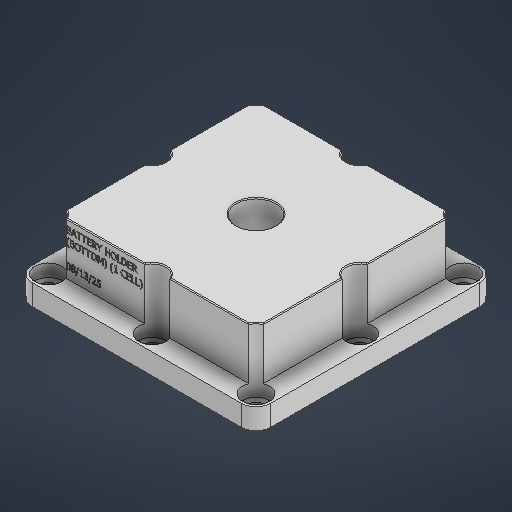
# Autodesk Inventor part: Battery Holder
Saved by Autodesk Inventor 2025 (Build 290162000, 162)
## iProperties
Created: 2025-08-08
Part Number: Battery Holder
Material: Generic
Document SubType Name: Modeling
Designer: mayhe
Density: 1 g/cm^3
Appearance: Default
Author: mayhe
Autodesk Inventor part; units mm, degrees
ref_plane "YZ Plane" through (0, 0, 0) normal (1, 0, 0) x (0, 1, 0)
ref_plane "XZ Plane" through (0, 0, 0) normal (0, 1, 0) x (-1, 0, 0)
ref_plane "XY Plane" through (0, 0, 0) normal (0, 0, 1) x (1, 0, 0)
sketch "Sketch1" plane through (0, 0, 0) normal (0, 1, 0) x (-1, 0, 0)
  line L0 (57.5, 57.5) -> (-57.5, 57.5)
  line L1 (-57.5, 57.5) -> (-57.5, -57.5)
  line L2 (-57.5, -57.5) -> (57.5, -57.5)
  line L3 (57.5, -57.5) -> (57.5, 57.5)
  line L4 (57.5, 57.5) -> (-57.5, -57.5) construction
  line L5 (-57.5, 57.5) -> (57.5, -57.5) construction
  point P0 (0, 0)
  dimension "d0" = 115
  dimension "d1" = 115
  constraints: 12 end point, 2 midpoint, 2 parallel, 1 horizontal, 1 perpendicular
  measures "d0" distance of L2.end L1.end
  measures "d1" distance of L1.end L0.end
extrude "Extrusion1" add sketch "Sketch1" along normal blind 10
sketch "Sketch4" plane through (0, 10, 0) normal (0, 1, 0) x (1, 0, 0)
  line L0 (-47.5, -47.5) -> (47.5, -47.5)
  line L1 (47.5, -47.5) -> (47.5, 47.5)
  line L2 (47.5, 47.5) -> (-47.5, 47.5)
  line L3 (-47.5, 47.5) -> (-47.5, -47.5)
  line L4 (-57.5, 57.5) -> (-57.5, -57.5) projected
  line L5 (-57.5, 0) -> (-47.5, 0)
  circle A0 centre (0, 0) radius 9.5
  point P0 (47.3285, -94.6135)
  point P1 (-53.5957, 219.1108)
  dimension "d48" = 95
  dimension "d49" = 95
  dimension "d180" = 19
  constraints: 10 end point, 2 midpoint, 2 parallel, 1 centre point, 1 horizontal, 1 perpendicular
  measures "d48" distance of L2.end L1.end
  measures "d49" distance of L1.end L0.end
  measures "d180" diameter of A0
extrude "Extrusion2" add sketch "Sketch4" along normal blind 25
sketch "Sketch5" plane through (0, 35, 0) normal (0, 1, 0) x (1, 0, 0)
  line L0 (50, 50) -> (-50, 50)
  line L1 (-50, 50) -> (-50, -50)
  line L2 (-50, -50) -> (50, -50)
  line L3 (50, -50) -> (50, 50)
  line L4 (50, 50) -> (-50, -50) construction
  line L5 (-50, 50) -> (50, -50) construction
  circle A0 centre (-50, -50) radius 3.5
  circle A1 centre (0, -50) radius 3.5
  circle A2 centre (-50, 0) radius 3.5
  circle A3 centre (0, 0) radius 3.5
  circle A4 centre (50, -50) radius 3.5
  circle A5 centre (50, 0) radius 3.5
  circle A6 centre (-50, 50) radius 3.5
  circle A7 centre (0, 50) radius 3.5
  circle A8 centre (50, 50) radius 3.5
  point P0 (0, 0)
  dimension "d156" = 100
  dimension "d157" = 100
  dimension "d158" = 7
  dimension "d161" = 50
  dimension "d164" = 50
  constraints: 12 end point, 9 centre point, 2 horizontal, 2 midpoint, 2 parallel, 1 coincident, 1 perpendicular, 1 vertical, 16 other
  measures "d156" distance of L2.end L1.end
  measures "d157" distance of L1.end L0.end
  measures "d158" diameter of A0
  measures "d161" distance of A0.centre A1.centre
  measures "d164" distance of A0.centre A2.centre
hole "Hole3" at (-50, 35, 50) at (50, 35, 50) at (-50, 35, -50) at (50, 35, -50) at (-50, 35, 0) at (0, 35, 50) at (50, 35, 0) at (0, 35, -50) direction (0, -1, 0) diameter 7.125 end through all counterbore diameter 13 counterbore depth 31
fillet "Fillet1" radius 7.125 4 edges at (57.5, 5, 57.5) (57.5, 5, -57.5) (-57.5, 5, 57.5) (-57.5, 5, -57.5)
chamfer "Chamfer1" distance 0.4 angle 45 18 edges at (-9.5, 35, 0) (-25, 35, 47.5) (0, 35, 43.5) (25, 35, 47.5) (47.5, 35, 25) (45.4038, 35, 45.4038) (43.5, 35, 0) (47.5, 35, -25) (45.4038, 35, -45.4038) (25, 35, -47.5) (3.6056, 35, -44.5917) (-3.6056, 35, -44.5917) (-25, 35, -47.5) (-45.4038, 35, -45.4038) (-47.5, 35, -25) (-43.5, 35, 0) (-47.5, 35, 25) (-45.4038, 35, 45.4038)
sketch "Sketch6" plane through (-44, 10, 47.5) normal (0, 0, 1) x (1, 0, 0)
  line L0 (0.0452, 22.2383) -> (37.6738, 22.2383) construction
  line L1 (37.6738, 22.2383) -> (37.6738, -2.1213) construction
  line L2 (37.6738, -2.1213) -> (0.0452, -2.1213) construction
  line L3 (0.0452, -2.1213) -> (0.0452, 22.2383) construction
  spline S0 degree 2 poles (2.4213, 20.0622) (2.4213, 19.835) (2.2484, 19.4867) (2.1052, 19.3731) knots 0 0 0 1 2 2 2
  spline S1 degree 2 poles (2.1052, 19.3731) (1.9323, 19.2397) (1.5395, 19.1261) (1.2283, 19.1261) knots 0 0 0 1 2 2 2
  line L4 (1.2283, 19.1261) -> (0.3539, 19.1261)
  line L5 (0.3539, 19.1261) -> (0.3539, 22.1741)
  line L6 (0.3539, 22.1741) -> (1.1616, 22.1741)
  spline S2 degree 2 poles (1.1616, 22.1741) (1.4877, 22.1741) (1.8137, 22.1321) (1.9619, 22.0506) knots 0 0 0 1 2 2 2
  spline S3 degree 2 poles (1.9619, 22.0506) (2.1274, 21.9641) (2.2781, 21.6801) (2.2781, 21.4874) knots 0 0 0 1 2 2 2
  spline S4 degree 2 poles (2.2781, 21.4874) (2.2781, 21.2725) (2.0508, 20.9316) (1.8507, 20.8353) knots 0 0 0 1 2 2 2
  line L7 (1.8507, 20.8353) -> (1.8507, 20.8205)
  spline S5 degree 2 poles (1.8507, 20.8205) (2.1224, 20.7464) (2.4213, 20.3537) (2.4213, 20.0622) knots 0 0 0 1 2 2 2
  spline S6 degree 2 poles (1.9989, 20.0449) (1.9989, 20.2178) (1.9001, 20.4401) (1.7519, 20.5191) knots 0 0 0 1 2 2 2
  spline S7 degree 2 poles (1.7519, 20.5191) (1.6556, 20.5685) (1.4284, 20.5982) (1.2184, 20.5982) knots 0 0 0 1 2 2 2
  line L8 (1.2184, 20.5982) -> (0.759, 20.5982)
  line L9 (0.759, 20.5982) -> (0.759, 19.4719)
  line L10 (0.759, 19.4719) -> (1.0875, 19.4719)
  spline S8 degree 2 poles (1.0875, 19.4719) (1.3543, 19.4719) (1.6606, 19.5213) (1.7791, 19.6003) knots 0 0 0 1 2 2 2
  spline S9 degree 2 poles (1.7791, 19.6003) (1.8927, 19.6818) (1.9989, 19.8844) (1.9989, 20.0449) knots 0 0 0 1 2 2 2
  spline S10 degree 2 poles (1.8557, 21.4306) (1.8557, 21.5393) (1.7816, 21.7023) (1.7001, 21.7492) knots 0 0 0 1 2 2 2
  spline S11 degree 2 poles (1.7001, 21.7492) (1.6013, 21.8036) (1.3617, 21.8283) (1.1468, 21.8283) knots 0 0 0 1 2 2 2
  line L11 (1.1468, 21.8283) -> (0.759, 21.8283)
  line L12 (0.759, 21.8283) -> (0.759, 20.9366)
  line L13 (0.759, 20.9366) -> (1.2184, 20.9366)
  spline S12 degree 2 poles (1.2184, 20.9366) (1.4086, 20.9366) (1.5889, 20.9761) (1.6853, 21.0378) knots 0 0 0 1 2 2 2
  spline S13 degree 2 poles (1.6853, 21.0378) (1.7791, 21.0971) (1.8557, 21.2873) (1.8557, 21.4306) knots 0 0 0 1 2 2 2
  line L14 (2.4954, 19.1261) -> (3.5229, 22.1741)
  line L15 (3.5229, 22.1741) -> (4.0219, 22.1741)
  line L16 (4.0219, 22.1741) -> (5.0494, 19.1261)
  line L17 (5.0494, 19.1261) -> (4.6221, 19.1261)
  line L18 (4.6221, 19.1261) -> (4.3455, 19.9782)
  line L19 (4.3455, 19.9782) -> (3.1821, 19.9782)
  line L20 (3.1821, 19.9782) -> (2.9054, 19.1261)
  line L21 (2.9054, 19.1261) -> (2.4954, 19.1261)
  line L22 (4.2343, 20.324) -> (3.7625, 21.7591)
  line L23 (3.7625, 21.7591) -> (3.2932, 20.324)
  line L24 (3.2932, 20.324) -> (4.2343, 20.324)
  line L25 (6.0498, 19.1261) -> (6.0498, 21.8134)
  line L26 (6.0498, 21.8134) -> (5.0272, 21.8134)
  line L27 (5.0272, 21.8134) -> (5.0272, 22.1741)
  line L28 (5.0272, 22.1741) -> (7.4774, 22.1741)
  line L29 (7.4774, 22.1741) -> (7.4774, 21.8134)
  line L30 (7.4774, 21.8134) -> (6.4549, 21.8134)
  line L31 (6.4549, 21.8134) -> (6.4549, 19.1261)
  line L32 (6.4549, 19.1261) -> (6.0498, 19.1261)
  line L33 (8.4976, 19.1261) -> (8.4976, 21.8134)
  line L34 (8.4976, 21.8134) -> (7.475, 21.8134)
  line L35 (7.475, 21.8134) -> (7.475, 22.1741)
  line L36 (7.475, 22.1741) -> (9.9252, 22.1741)
  line L37 (9.9252, 22.1741) -> (9.9252, 21.8134)
  line L38 (9.9252, 21.8134) -> (8.9026, 21.8134)
  line L39 (8.9026, 21.8134) -> (8.9026, 19.1261)
  line L40 (8.9026, 19.1261) -> (8.4976, 19.1261)
  line L41 (10.234, 19.1261) -> (10.234, 22.1741)
  line L42 (10.234, 22.1741) -> (12.1408, 22.1741)
  line L43 (12.1408, 22.1741) -> (12.1408, 21.8134)
  line L44 (12.1408, 21.8134) -> (10.6391, 21.8134)
  line L45 (10.6391, 21.8134) -> (10.6391, 20.9786)
  line L46 (10.6391, 20.9786) -> (12.0396, 20.9786)
  line L47 (12.0396, 20.9786) -> (12.0396, 20.6179)
  line L48 (12.0396, 20.6179) -> (10.6391, 20.6179)
  line L49 (10.6391, 20.6179) -> (10.6391, 19.4867)
  line L50 (10.6391, 19.4867) -> (12.1408, 19.4867)
  line L51 (12.1408, 19.4867) -> (12.1408, 19.1261)
  line L52 (12.1408, 19.1261) -> (10.234, 19.1261)
  line L53 (14.9443, 19.1261) -> (14.4182, 19.1261)
  line L54 (14.4182, 19.1261) -> (13.4549, 20.3388)
  line L55 (13.4549, 20.3388) -> (12.9905, 20.3388)
  line L56 (12.9905, 20.3388) -> (12.9905, 19.1261)
  line L57 (12.9905, 19.1261) -> (12.5854, 19.1261)
  line L58 (12.5854, 19.1261) -> (12.5854, 22.1741)
  line L59 (12.5854, 22.1741) -> (13.3709, 22.1741)
  spline S14 degree 2 poles (13.3709, 22.1741) (13.6327, 22.1741) (13.9859, 22.1172) (14.1465, 22.0135) knots 0 0 0 1 2 2 2
  spline S15 degree 2 poles (14.1465, 22.0135) (14.307, 21.9098) (14.4923, 21.5862) (14.4923, 21.3466) knots 0 0 0 1 2 2 2
  spline S16 degree 2 poles (14.4923, 21.3466) (14.4923, 21.0131) (14.1514, 20.5611) (13.86, 20.4525) knots 0 0 0 1 2 2 2
  line L60 (13.86, 20.4525) -> (14.9443, 19.1261)
  spline S17 degree 2 poles (14.0699, 21.3145) (14.0699, 21.4479) (13.9761, 21.6529) (13.8773, 21.7196) knots 0 0 0 1 2 2 2
  spline S18 degree 2 poles (13.8773, 21.7196) (13.7908, 21.7764) (13.5611, 21.8233) (13.3931, 21.8233) knots 0 0 0 1 2 2 2
  line L61 (13.3931, 21.8233) -> (12.9905, 21.8233)
  line L62 (12.9905, 21.8233) -> (12.9905, 20.6772)
  line L63 (12.9905, 20.6772) -> (13.3462, 20.6772)
  spline S19 degree 2 poles (13.3462, 20.6772) (13.5216, 20.6772) (13.8007, 20.739) (13.897, 20.8353) knots 0 0 0 1 2 2 2
  spline S20 degree 2 poles (13.897, 20.8353) (13.9859, 20.9193) (14.0699, 21.1564) (14.0699, 21.3145) knots 0 0 0 1 2 2 2
  line L64 (17.3205, 22.1741) -> (16.2905, 20.4747)
  line L65 (16.2905, 20.4747) -> (16.2905, 19.1261)
  line L66 (16.2905, 19.1261) -> (15.8854, 19.1261)
  line L67 (15.8854, 19.1261) -> (15.8854, 20.4327)
  line L68 (15.8854, 20.4327) -> (14.8554, 22.1741)
  line L69 (14.8554, 22.1741) -> (15.3049, 22.1741)
  line L70 (15.3049, 22.1741) -> (16.0929, 20.8328)
  line L71 (16.0929, 20.8328) -> (16.8907, 22.1741)
  line L72 (16.8907, 22.1741) -> (17.3205, 22.1741)
  line L73 (21.1243, 19.1261) -> (20.7192, 19.1261)
  line L74 (20.7192, 19.1261) -> (20.7192, 20.6179)
  line L75 (20.7192, 20.6179) -> (19.3162, 20.6179)
  line L76 (19.3162, 20.6179) -> (19.3162, 19.1261)
  line L77 (19.3162, 19.1261) -> (18.9111, 19.1261)
  line L78 (18.9111, 19.1261) -> (18.9111, 22.1741)
  line L79 (18.9111, 22.1741) -> (19.3162, 22.1741)
  line L80 (19.3162, 22.1741) -> (19.3162, 20.9786)
  line L81 (19.3162, 20.9786) -> (20.7192, 20.9786)
  line L82 (20.7192, 20.9786) -> (20.7192, 22.1741)
  line L83 (20.7192, 22.1741) -> (21.1243, 22.1741)
  line L84 (21.1243, 22.1741) -> (21.1243, 19.1261)
  spline S21 degree 2 poles (23.8981, 21.8258) (24.071, 21.6232) (24.2637, 21.0304) (24.2637, 20.6501) knots 0 0 0 1 2 2 2
  spline S22 degree 2 poles (24.2637, 20.6501) (24.2637, 20.2796) (24.076, 19.6793) (23.8981, 19.4768) knots 0 0 0 1 2 2 2
  spline S23 degree 2 poles (23.8981, 19.4768) (23.7104, 19.2644) (23.2139, 19.0618) (22.915, 19.0618) knots 0 0 0 1 2 2 2
  spline S24 degree 2 poles (22.915, 19.0618) (22.6063, 19.0618) (22.1123, 19.2718) (21.932, 19.4768) knots 0 0 0 1 2 2 2
  spline S25 degree 2 poles (21.932, 19.4768) (21.7566, 19.6793) (21.5689, 20.2746) (21.5689, 20.6501) knots 0 0 0 1 2 2 2
  spline S26 degree 2 poles (21.5689, 20.6501) (21.5689, 21.0329) (21.7591, 21.6158) (21.9344, 21.8258) knots 0 0 0 1 2 2 2
  spline S27 degree 2 poles (21.9344, 21.8258) (22.1123, 22.0283) (22.6088, 22.2383) (22.915, 22.2383) knots 0 0 0 1 2 2 2
  spline S28 degree 2 poles (22.915, 22.2383) (23.2263, 22.2383) (23.7252, 22.0209) (23.8981, 21.8258) knots 0 0 0 1 2 2 2
  spline S29 degree 2 poles (23.8413, 20.6501) (23.8413, 20.9514) (23.7104, 21.4182) (23.5918, 21.5714) knots 0 0 0 1 2 2 2
  spline S30 degree 2 poles (23.5918, 21.5714) (23.4708, 21.7295) (23.1299, 21.8875) (22.9175, 21.8875) knots 0 0 0 1 2 2 2
  spline S31 degree 2 poles (22.9175, 21.8875) (22.6977, 21.8875) (22.3667, 21.7344) (22.2407, 21.5714) knots 0 0 0 1 2 2 2
  spline S32 degree 2 poles (22.2407, 21.5714) (22.1197, 21.4158) (21.9913, 20.9465) (21.9913, 20.6501) knots 0 0 0 1 2 2 2
  spline S33 degree 2 poles (21.9913, 20.6501) (21.9913, 20.0498) (22.4951, 19.4126) (22.9175, 19.4126) knots 0 0 0 1 2 2 2
  spline S34 degree 2 poles (22.9175, 19.4126) (23.3399, 19.4126) (23.8413, 20.0498) (23.8413, 20.6501) knots 0 0 0 1 2 2 2
  line L85 (26.4743, 19.1261) -> (24.7083, 19.1261)
  line L86 (24.7083, 19.1261) -> (24.7083, 22.1741)
  line L87 (24.7083, 22.1741) -> (25.1134, 22.1741)
  line L88 (25.1134, 22.1741) -> (25.1134, 19.4867)
  line L89 (25.1134, 19.4867) -> (26.4743, 19.4867)
  line L90 (26.4743, 19.4867) -> (26.4743, 19.1261)
  spline S35 degree 2 poles (29.1963, 20.6476) (29.1963, 20.2302) (28.8579, 19.5583) (28.5739, 19.3706) knots 0 0 0 1 2 2 2
  spline S36 degree 2 poles (28.5739, 19.3706) (28.3417, 19.2249) (27.865, 19.1261) (27.4945, 19.1261) knots 0 0 0 1 2 2 2
  line L91 (27.4945, 19.1261) -> (26.793, 19.1261)
  line L92 (26.793, 19.1261) -> (26.793, 22.1741)
  line L93 (26.793, 22.1741) -> (27.487, 22.1741)
  spline S37 degree 2 poles (27.487, 22.1741) (27.9168, 22.1741) (28.4059, 22.0456) (28.5788, 21.932) knots 0 0 0 1 2 2 2
  spline S38 degree 2 poles (28.5788, 21.932) (28.8727, 21.7369) (29.1963, 21.0922) (29.1963, 20.6476) knots 0 0 0 1 2 2 2
  spline S39 degree 2 poles (28.7739, 20.6525) (28.7739, 21.0033) (28.5417, 21.4997) (28.312, 21.6405) knots 0 0 0 1 2 2 2
  spline S40 degree 2 poles (28.312, 21.6405) (28.149, 21.7369) (27.781, 21.8233) (27.5068, 21.8233) knots 0 0 0 1 2 2 2
  line L94 (27.5068, 21.8233) -> (27.1981, 21.8233)
  line L95 (27.1981, 21.8233) -> (27.1981, 19.4768)
  line L96 (27.1981, 19.4768) -> (27.5068, 19.4768)
  spline S41 degree 2 poles (27.5068, 19.4768) (27.776, 19.4768) (28.1836, 19.5632) (28.3491, 19.6793) knots 0 0 0 1 2 2 2
  spline S42 degree 2 poles (28.3491, 19.6793) (28.5615, 19.8226) (28.7739, 20.2968) (28.7739, 20.6525) knots 0 0 0 1 2 2 2
  line L97 (29.636, 19.1261) -> (29.636, 22.1741)
  line L98 (29.636, 22.1741) -> (31.5428, 22.1741)
  line L99 (31.5428, 22.1741) -> (31.5428, 21.8134)
  line L100 (31.5428, 21.8134) -> (30.041, 21.8134)
  line L101 (30.041, 21.8134) -> (30.041, 20.9786)
  line L102 (30.041, 20.9786) -> (31.4415, 20.9786)
  line L103 (31.4415, 20.9786) -> (31.4415, 20.6179)
  line L104 (31.4415, 20.6179) -> (30.041, 20.6179)
  line L105 (30.041, 20.6179) -> (30.041, 19.4867)
  line L106 (30.041, 19.4867) -> (31.5428, 19.4867)
  line L107 (31.5428, 19.4867) -> (31.5428, 19.1261)
  line L108 (31.5428, 19.1261) -> (29.636, 19.1261)
  line L109 (34.3463, 19.1261) -> (33.8202, 19.1261)
  line L110 (33.8202, 19.1261) -> (32.8569, 20.3388)
  line L111 (32.8569, 20.3388) -> (32.3925, 20.3388)
  line L112 (32.3925, 20.3388) -> (32.3925, 19.1261)
  line L113 (32.3925, 19.1261) -> (31.9874, 19.1261)
  line L114 (31.9874, 19.1261) -> (31.9874, 22.1741)
  line L115 (31.9874, 22.1741) -> (32.7729, 22.1741)
  spline S43 degree 2 poles (32.7729, 22.1741) (33.0347, 22.1741) (33.3879, 22.1172) (33.5485, 22.0135) knots 0 0 0 1 2 2 2
  spline S44 degree 2 poles (33.5485, 22.0135) (33.709, 21.9098) (33.8943, 21.5862) (33.8943, 21.3466) knots 0 0 0 1 2 2 2
  spline S45 degree 2 poles (33.8943, 21.3466) (33.8943, 21.0131) (33.5534, 20.5611) (33.2619, 20.4525) knots 0 0 0 1 2 2 2
  line L116 (33.2619, 20.4525) -> (34.3463, 19.1261)
  spline S46 degree 2 poles (33.4719, 21.3145) (33.4719, 21.4479) (33.378, 21.6529) (33.2792, 21.7196) knots 0 0 0 1 2 2 2
  spline S47 degree 2 poles (33.2792, 21.7196) (33.1928, 21.7764) (32.9631, 21.8233) (32.7951, 21.8233) knots 0 0 0 1 2 2 2
  line L117 (32.7951, 21.8233) -> (32.3925, 21.8233)
  line L118 (32.3925, 21.8233) -> (32.3925, 20.6772)
  line L119 (32.3925, 20.6772) -> (32.7482, 20.6772)
  spline S48 degree 2 poles (32.7482, 20.6772) (32.9235, 20.6772) (33.2027, 20.739) (33.299, 20.8353) knots 0 0 0 1 2 2 2
  spline S49 degree 2 poles (33.299, 20.8353) (33.3879, 20.9193) (33.4719, 21.1564) (33.4719, 21.3145) knots 0 0 0 1 2 2 2
  line L120 (1.4975, 13.2653) -> (1.0282, 13.2653)
  spline S50 degree 2 poles (1.0282, 13.2653) (0.6725, 13.6877) (0.265, 14.6337) (0.265, 15.2784) knots 0 0 0 1 2 2 2
  spline S51 degree 2 poles (0.265, 15.2784) (0.265, 15.9082) (0.6676, 16.8691) (1.0282, 17.2915) knots 0 0 0 1 2 2 2
  line L121 (1.0282, 17.2915) -> (1.4975, 17.2915)
  line L122 (1.4975, 17.2915) -> (1.4975, 17.2717)
  spline S52 degree 2 poles (1.4975, 17.2717) (1.332, 17.121) (1.0307, 16.7308) (0.9023, 16.4714) knots 0 0 0 1 2 2 2
  spline S53 degree 2 poles (0.9023, 16.4714) (0.7788, 16.2195) (0.6256, 15.6143) (0.6256, 15.2784) knots 0 0 0 1 2 2 2
  spline S54 degree 2 poles (0.6256, 15.2784) (0.6256, 14.9276) (0.7738, 14.3472) (0.9023, 14.0854) knots 0 0 0 1 2 2 2
  spline S55 degree 2 poles (0.9023, 14.0854) (1.0258, 13.8334) (1.3395, 13.4259) (1.4975, 13.2851) knots 0 0 0 1 2 2 2
  line L123 (1.4975, 13.2851) -> (1.4975, 13.2653)
  spline S56 degree 2 poles (4.0268, 15.0437) (4.0268, 14.8165) (3.8539, 14.4682) (3.7107, 14.3546) knots 0 0 0 1 2 2 2
  spline S57 degree 2 poles (3.7107, 14.3546) (3.5378, 14.2212) (3.145, 14.1076) (2.8338, 14.1076) knots 0 0 0 1 2 2 2
  line L124 (2.8338, 14.1076) -> (1.9594, 14.1076)
  line L125 (1.9594, 14.1076) -> (1.9594, 17.1556)
  line L126 (1.9594, 17.1556) -> (2.7671, 17.1556)
  spline S58 degree 2 poles (2.7671, 17.1556) (3.0932, 17.1556) (3.4192, 17.1136) (3.5674, 17.0321) knots 0 0 0 1 2 2 2
  spline S59 degree 2 poles (3.5674, 17.0321) (3.7329, 16.9457) (3.8836, 16.6616) (3.8836, 16.4689) knots 0 0 0 1 2 2 2
  spline S60 degree 2 poles (3.8836, 16.4689) (3.8836, 16.254) (3.6563, 15.9132) (3.4563, 15.8169) knots 0 0 0 1 2 2 2
  line L127 (3.4563, 15.8169) -> (3.4563, 15.802)
  spline S61 degree 2 poles (3.4563, 15.802) (3.728, 15.7279) (4.0268, 15.3352) (4.0268, 15.0437) knots 0 0 0 1 2 2 2
  spline S62 degree 2 poles (3.6045, 15.0265) (3.6045, 15.1994) (3.5057, 15.4217) (3.3575, 15.5007) knots 0 0 0 1 2 2 2
  spline S63 degree 2 poles (3.3575, 15.5007) (3.2611, 15.5501) (3.0339, 15.5797) (2.8239, 15.5797) knots 0 0 0 1 2 2 2
  line L128 (2.8239, 15.5797) -> (2.3645, 15.5797)
  line L129 (2.3645, 15.5797) -> (2.3645, 14.4534)
  line L130 (2.3645, 14.4534) -> (2.693, 14.4534)
  spline S64 degree 2 poles (2.693, 14.4534) (2.9598, 14.4534) (3.2661, 14.5028) (3.3846, 14.5818) knots 0 0 0 1 2 2 2
  spline S65 degree 2 poles (3.3846, 14.5818) (3.4982, 14.6634) (3.6045, 14.8659) (3.6045, 15.0265) knots 0 0 0 1 2 2 2
  spline S66 degree 2 poles (3.4612, 16.4121) (3.4612, 16.5208) (3.3871, 16.6838) (3.3056, 16.7308) knots 0 0 0 1 2 2 2
  spline S67 degree 2 poles (3.3056, 16.7308) (3.2068, 16.7851) (2.9672, 16.8098) (2.7523, 16.8098) knots 0 0 0 1 2 2 2
  line L131 (2.7523, 16.8098) -> (2.3645, 16.8098)
  line L132 (2.3645, 16.8098) -> (2.3645, 15.9181)
  line L133 (2.3645, 15.9181) -> (2.8239, 15.9181)
  spline S68 degree 2 poles (2.8239, 15.9181) (3.0141, 15.9181) (3.1944, 15.9576) (3.2908, 16.0194) knots 0 0 0 1 2 2 2
  spline S69 degree 2 poles (3.2908, 16.0194) (3.3846, 16.0787) (3.4612, 16.2689) (3.4612, 16.4121) knots 0 0 0 1 2 2 2
  spline S70 degree 2 poles (6.5858, 16.8073) (6.7587, 16.6048) (6.9513, 16.012) (6.9513, 15.6316) knots 0 0 0 1 2 2 2
  spline S71 degree 2 poles (6.9513, 15.6316) (6.9513, 15.2611) (6.7636, 14.6609) (6.5858, 14.4583) knots 0 0 0 1 2 2 2
  spline S72 degree 2 poles (6.5858, 14.4583) (6.398, 14.2459) (5.9016, 14.0434) (5.6027, 14.0434) knots 0 0 0 1 2 2 2
  spline S73 degree 2 poles (5.6027, 14.0434) (5.2939, 14.0434) (4.7999, 14.2533) (4.6196, 14.4583) knots 0 0 0 1 2 2 2
  spline S74 degree 2 poles (4.6196, 14.4583) (4.4443, 14.6609) (4.2565, 15.2562) (4.2565, 15.6316) knots 0 0 0 1 2 2 2
  spline S75 degree 2 poles (4.2565, 15.6316) (4.2565, 16.0145) (4.4467, 16.5974) (4.6221, 16.8073) knots 0 0 0 1 2 2 2
  spline S76 degree 2 poles (4.6221, 16.8073) (4.7999, 17.0099) (5.2964, 17.2198) (5.6027, 17.2198) knots 0 0 0 1 2 2 2
  spline S77 degree 2 poles (5.6027, 17.2198) (5.9139, 17.2198) (6.4129, 17.0025) (6.5858, 16.8073) knots 0 0 0 1 2 2 2
  spline S78 degree 2 poles (6.529, 15.6316) (6.529, 15.9329) (6.398, 16.3998) (6.2795, 16.5529) knots 0 0 0 1 2 2 2
  spline S79 degree 2 poles (6.2795, 16.5529) (6.1585, 16.711) (5.8176, 16.8691) (5.6052, 16.8691) knots 0 0 0 1 2 2 2
  spline S80 degree 2 poles (5.6052, 16.8691) (5.3853, 16.8691) (5.0544, 16.7159) (4.9284, 16.5529) knots 0 0 0 1 2 2 2
  spline S81 degree 2 poles (4.9284, 16.5529) (4.8074, 16.3973) (4.6789, 15.928) (4.6789, 15.6316) knots 0 0 0 1 2 2 2
  spline S82 degree 2 poles (4.6789, 15.6316) (4.6789, 15.0314) (5.1828, 14.3941) (5.6052, 14.3941) knots 0 0 0 1 2 2 2
  spline S83 degree 2 poles (5.6052, 14.3941) (6.0275, 14.3941) (6.529, 15.0314) (6.529, 15.6316) knots 0 0 0 1 2 2 2
  line L134 (8.1073, 14.1076) -> (8.1073, 16.795)
  line L135 (8.1073, 16.795) -> (7.0847, 16.795)
  line L136 (7.0847, 16.795) -> (7.0847, 17.1556)
  line L137 (7.0847, 17.1556) -> (9.535, 17.1556)
  line L138 (9.535, 17.1556) -> (9.535, 16.795)
  line L139 (9.535, 16.795) -> (8.5124, 16.795)
  line L140 (8.5124, 16.795) -> (8.5124, 14.1076)
  line L141 (8.5124, 14.1076) -> (8.1073, 14.1076)
  line L142 (10.5551, 14.1076) -> (10.5551, 16.795)
  line L143 (10.5551, 16.795) -> (9.5325, 16.795)
  line L144 (9.5325, 16.795) -> (9.5325, 17.1556)
  line L145 (9.5325, 17.1556) -> (11.9828, 17.1556)
  line L146 (11.9828, 17.1556) -> (11.9828, 16.795)
  line L147 (11.9828, 16.795) -> (10.9602, 16.795)
  line L148 (10.9602, 16.795) -> (10.9602, 14.1076)
  line L149 (10.9602, 14.1076) -> (10.5551, 14.1076)
  spline S84 degree 2 poles (14.4478, 16.8073) (14.6207, 16.6048) (14.8134, 16.012) (14.8134, 15.6316) knots 0 0 0 1 2 2 2
  spline S85 degree 2 poles (14.8134, 15.6316) (14.8134, 15.2611) (14.6257, 14.6609) (14.4478, 14.4583) knots 0 0 0 1 2 2 2
  spline S86 degree 2 poles (14.4478, 14.4583) (14.2601, 14.2459) (13.7636, 14.0434) (13.4648, 14.0434) knots 0 0 0 1 2 2 2
  spline S87 degree 2 poles (13.4648, 14.0434) (13.156, 14.0434) (12.662, 14.2533) (12.4817, 14.4583) knots 0 0 0 1 2 2 2
  spline S88 degree 2 poles (12.4817, 14.4583) (12.3063, 14.6609) (12.1186, 15.2562) (12.1186, 15.6316) knots 0 0 0 1 2 2 2
  spline S89 degree 2 poles (12.1186, 15.6316) (12.1186, 16.0145) (12.3088, 16.5974) (12.4842, 16.8073) knots 0 0 0 1 2 2 2
  spline S90 degree 2 poles (12.4842, 16.8073) (12.662, 17.0099) (13.1585, 17.2198) (13.4648, 17.2198) knots 0 0 0 1 2 2 2
  spline S91 degree 2 poles (13.4648, 17.2198) (13.776, 17.2198) (14.2749, 17.0025) (14.4478, 16.8073) knots 0 0 0 1 2 2 2
  spline S92 degree 2 poles (14.391, 15.6316) (14.391, 15.9329) (14.2601, 16.3998) (14.1415, 16.5529) knots 0 0 0 1 2 2 2
  spline S93 degree 2 poles (14.1415, 16.5529) (14.0205, 16.711) (13.6797, 16.8691) (13.4672, 16.8691) knots 0 0 0 1 2 2 2
  spline S94 degree 2 poles (13.4672, 16.8691) (13.2474, 16.8691) (12.9164, 16.7159) (12.7904, 16.5529) knots 0 0 0 1 2 2 2
  spline S95 degree 2 poles (12.7904, 16.5529) (12.6694, 16.3973) (12.541, 15.928) (12.541, 15.6316) knots 0 0 0 1 2 2 2
  spline S96 degree 2 poles (12.541, 15.6316) (12.541, 15.0314) (13.0449, 14.3941) (13.4672, 14.3941) knots 0 0 0 1 2 2 2
  spline S97 degree 2 poles (13.4672, 14.3941) (13.8896, 14.3941) (14.391, 15.0314) (14.391, 15.6316) knots 0 0 0 1 2 2 2
  line L150 (17.8713, 14.1076) -> (17.4662, 14.1076)
  line L151 (17.4662, 14.1076) -> (17.4662, 16.7332)
  line L152 (17.4662, 16.7332) -> (16.6708, 14.9474)
  line L153 (16.6708, 14.9474) -> (16.4238, 14.9474)
  line L154 (16.4238, 14.9474) -> (15.6359, 16.7332)
  line L155 (15.6359, 16.7332) -> (15.6359, 14.1076)
  line L156 (15.6359, 14.1076) -> (15.258, 14.1076)
  line L157 (15.258, 14.1076) -> (15.258, 17.1556)
  line L158 (15.258, 17.1556) -> (15.8113, 17.1556)
  line L159 (15.8113, 17.1556) -> (16.572, 15.4587)
  line L160 (16.572, 15.4587) -> (17.3081, 17.1556)
  line L161 (17.3081, 17.1556) -> (17.8713, 17.1556)
  line L162 (17.8713, 17.1556) -> (17.8713, 14.1076)
  spline S98 degree 2 poles (19.5657, 15.2784) (19.5657, 14.6461) (19.1606, 13.6877) (18.8025, 13.2653) knots 0 0 0 1 2 2 2
  line L163 (18.8025, 13.2653) -> (18.3332, 13.2653)
  line L164 (18.3332, 13.2653) -> (18.3332, 13.2851)
  spline S99 degree 2 poles (18.3332, 13.2851) (18.4912, 13.4259) (18.8099, 13.8384) (18.9284, 14.0854) knots 0 0 0 1 2 2 2
  spline S100 degree 2 poles (18.9284, 14.0854) (19.0569, 14.3497) (19.2051, 14.9375) (19.2051, 15.2784) knots 0 0 0 1 2 2 2
  spline S101 degree 2 poles (19.2051, 15.2784) (19.2051, 15.6168) (19.0544, 16.217) (18.9284, 16.4714) knots 0 0 0 1 2 2 2
  spline S102 degree 2 poles (18.9284, 16.4714) (18.8049, 16.7258) (18.4888, 17.1309) (18.3332, 17.2717) knots 0 0 0 1 2 2 2
  line L165 (18.3332, 17.2717) -> (18.3332, 17.2915)
  line L166 (18.3332, 17.2915) -> (18.8025, 17.2915)
  spline S103 degree 2 poles (18.8025, 17.2915) (19.1581, 16.8691) (19.5657, 15.9157) (19.5657, 15.2784) knots 0 0 0 1 2 2 2
  line L167 (22.547, 13.2653) -> (22.0777, 13.2653)
  spline S104 degree 2 poles (22.0777, 13.2653) (21.722, 13.6877) (21.3145, 14.6337) (21.3145, 15.2784) knots 0 0 0 1 2 2 2
  spline S105 degree 2 poles (21.3145, 15.2784) (21.3145, 15.9082) (21.7171, 16.8691) (22.0777, 17.2915) knots 0 0 0 1 2 2 2
  line L168 (22.0777, 17.2915) -> (22.547, 17.2915)
  line L169 (22.547, 17.2915) -> (22.547, 17.2717)
  spline S106 degree 2 poles (22.547, 17.2717) (22.3815, 17.121) (22.0802, 16.7308) (21.9517, 16.4714) knots 0 0 0 1 2 2 2
  spline S107 degree 2 poles (21.9517, 16.4714) (21.8282, 16.2195) (21.6751, 15.6143) (21.6751, 15.2784) knots 0 0 0 1 2 2 2
  spline S108 degree 2 poles (21.6751, 15.2784) (21.6751, 14.9276) (21.8233, 14.3472) (21.9517, 14.0854) knots 0 0 0 1 2 2 2
  spline S109 degree 2 poles (21.9517, 14.0854) (22.0752, 13.8334) (22.3889, 13.4259) (22.547, 13.2851) knots 0 0 0 1 2 2 2
  line L170 (22.547, 13.2851) -> (22.547, 13.2653)
  line L171 (24.649, 14.1076) -> (23.162, 14.1076)
  line L172 (23.162, 14.1076) -> (23.162, 14.4188)
  line L173 (23.162, 14.4188) -> (23.7153, 14.4188)
  line L174 (23.7153, 14.4188) -> (23.7153, 16.4615)
  line L175 (23.7153, 16.4615) -> (23.162, 16.4615)
  line L176 (23.162, 16.4615) -> (23.162, 16.7406)
  spline S110 degree 2 poles (23.162, 16.7406) (23.4757, 16.7406) (23.7721, 16.9185) (23.7919, 17.1655) knots 0 0 0 1 2 2 2
  line L177 (23.7919, 17.1655) -> (24.1081, 17.1655)
  line L178 (24.1081, 17.1655) -> (24.1081, 14.4188)
  line L179 (24.1081, 14.4188) -> (24.649, 14.4188)
  line L180 (24.649, 14.4188) -> (24.649, 14.1076)
  spline S111 degree 2 poles (27.7958, 14.0533) (27.4994, 14.0533) (26.998, 14.2533) (26.8152, 14.4534) knots 0 0 0 1 2 2 2
  spline S112 degree 2 poles (26.8152, 14.4534) (26.6324, 14.651) (26.4323, 15.2438) (26.4323, 15.6291) knots 0 0 0 1 2 2 2
  spline S113 degree 2 poles (26.4323, 15.6291) (26.4323, 16.012) (26.6275, 16.5801) (26.8127, 16.79) knots 0 0 0 1 2 2 2
  spline S114 degree 2 poles (26.8127, 16.79) (26.9955, 16.9951) (27.4945, 17.2099) (27.8032, 17.2099) knots 0 0 0 1 2 2 2
  spline S115 degree 2 poles (27.8032, 17.2099) (27.9563, 17.2099) (28.2256, 17.1655) (28.3392, 17.1309) knots 0 0 0 1 2 2 2
  spline S116 degree 2 poles (28.3392, 17.1309) (28.438, 17.0988) (28.643, 17.0074) (28.7443, 16.9531) knots 0 0 0 1 2 2 2
  line L181 (28.7443, 16.9531) -> (28.7443, 16.464)
  line L182 (28.7443, 16.464) -> (28.7122, 16.464)
  spline S117 degree 2 poles (28.7122, 16.464) (28.6578, 16.5134) (28.4899, 16.6517) (28.3688, 16.7184) knots 0 0 0 1 2 2 2
  spline S118 degree 2 poles (28.3688, 16.7184) (28.2527, 16.7826) (27.9786, 16.8641) (27.8007, 16.8641) knots 0 0 0 1 2 2 2
  spline S119 degree 2 poles (27.8007, 16.8641) (27.6056, 16.8641) (27.2573, 16.7036) (27.1264, 16.5505) knots 0 0 0 1 2 2 2
  spline S120 degree 2 poles (27.1264, 16.5505) (26.998, 16.3948) (26.8547, 15.9231) (26.8547, 15.6291) knots 0 0 0 1 2 2 2
  spline S121 degree 2 poles (26.8547, 15.6291) (26.8547, 15.3154) (27.0054, 14.8634) (27.1363, 14.7078) knots 0 0 0 1 2 2 2
  spline S122 degree 2 poles (27.1363, 14.7078) (27.2647, 14.5571) (27.6081, 14.404) (27.8007, 14.404) knots 0 0 0 1 2 2 2
  spline S123 degree 2 poles (27.8007, 14.404) (27.9761, 14.404) (28.275, 14.4905) (28.3911, 14.5547) knots 0 0 0 1 2 2 2
  spline S124 degree 2 poles (28.3911, 14.5547) (28.5022, 14.6189) (28.6677, 14.7523) (28.7146, 14.7992) knots 0 0 0 1 2 2 2
  line L183 (28.7146, 14.7992) -> (28.7443, 14.7992)
  line L184 (28.7443, 14.7992) -> (28.7443, 14.3151)
  spline S125 degree 2 poles (28.7443, 14.3151) (28.643, 14.2682) (28.4652, 14.1817) (28.3392, 14.1422) knots 0 0 0 1 2 2 2
  spline S126 degree 2 poles (28.3392, 14.1422) (28.2058, 14.0977) (27.9786, 14.0533) (27.7958, 14.0533) knots 0 0 0 1 2 2 2
  line L185 (29.1222, 14.1076) -> (29.1222, 17.1556)
  line L186 (29.1222, 17.1556) -> (31.029, 17.1556)
  line L187 (31.029, 17.1556) -> (31.029, 16.795)
  line L188 (31.029, 16.795) -> (29.5273, 16.795)
  line L189 (29.5273, 16.795) -> (29.5273, 15.9601)
  line L190 (29.5273, 15.9601) -> (30.9278, 15.9601)
  line L191 (30.9278, 15.9601) -> (30.9278, 15.5995)
  line L192 (30.9278, 15.5995) -> (29.5273, 15.5995)
  line L193 (29.5273, 15.5995) -> (29.5273, 14.4682)
  line L194 (29.5273, 14.4682) -> (31.029, 14.4682)
  line L195 (31.029, 14.4682) -> (31.029, 14.1076)
  line L196 (31.029, 14.1076) -> (29.1222, 14.1076)
  line L197 (33.2397, 14.1076) -> (31.4737, 14.1076)
  line L198 (31.4737, 14.1076) -> (31.4737, 17.1556)
  line L199 (31.4737, 17.1556) -> (31.8787, 17.1556)
  line L200 (31.8787, 17.1556) -> (31.8787, 14.4682)
  line L201 (31.8787, 14.4682) -> (33.2397, 14.4682)
  line L202 (33.2397, 14.4682) -> (33.2397, 14.1076)
  line L203 (35.3244, 14.1076) -> (33.5583, 14.1076)
  line L204 (33.5583, 14.1076) -> (33.5583, 17.1556)
  line L205 (33.5583, 17.1556) -> (33.9634, 17.1556)
  line L206 (33.9634, 17.1556) -> (33.9634, 14.4682)
  line L207 (33.9634, 14.4682) -> (35.3244, 14.4682)
  line L208 (35.3244, 14.4682) -> (35.3244, 14.1076)
  spline S127 degree 2 poles (36.72, 15.2784) (36.72, 14.6461) (36.3149, 13.6877) (35.9567, 13.2653) knots 0 0 0 1 2 2 2
  line L209 (35.9567, 13.2653) -> (35.4874, 13.2653)
  line L210 (35.4874, 13.2653) -> (35.4874, 13.2851)
  spline S128 degree 2 poles (35.4874, 13.2851) (35.6455, 13.4259) (35.9641, 13.8384) (36.0827, 14.0854) knots 0 0 0 1 2 2 2
  spline S129 degree 2 poles (36.0827, 14.0854) (36.2111, 14.3497) (36.3593, 14.9375) (36.3593, 15.2784) knots 0 0 0 1 2 2 2
  spline S130 degree 2 poles (36.3593, 15.2784) (36.3593, 15.6168) (36.2087, 16.217) (36.0827, 16.4714) knots 0 0 0 1 2 2 2
  spline S131 degree 2 poles (36.0827, 16.4714) (35.9592, 16.7258) (35.643, 17.1309) (35.4874, 17.2717) knots 0 0 0 1 2 2 2
  line L211 (35.4874, 17.2717) -> (35.4874, 17.2915)
  line L212 (35.4874, 17.2915) -> (35.9567, 17.2915)
  spline S132 degree 2 poles (35.9567, 17.2915) (36.3124, 16.8691) (36.72, 15.9157) (36.72, 15.2784) knots 0 0 0 1 2 2 2
  spline S133 degree 2 poles (2.1644, 5.5947) (2.1644, 4.7747) (1.6877, 4.0065) (1.1913, 4.0065) knots 0 0 0 1 2 2 2
  spline S134 degree 2 poles (1.1913, 4.0065) (0.6874, 4.0065) (0.2156, 4.7895) (0.2156, 5.5922) knots 0 0 0 1 2 2 2
  spline S135 degree 2 poles (0.2156, 5.5922) (0.2156, 6.4172) (0.6923, 7.1805) (1.1913, 7.1805) knots 0 0 0 1 2 2 2
  spline S136 degree 2 poles (1.1913, 7.1805) (1.6927, 7.1805) (2.1644, 6.39) (2.1644, 5.5947) knots 0 0 0 1 2 2 2
  spline S137 degree 2 poles (1.6408, 4.666) (1.7001, 4.8166) (1.7495, 5.281) (1.7495, 5.5947) knots 0 0 0 1 2 2 2
  spline S138 degree 2 poles (1.7495, 5.5947) (1.7495, 5.9084) (1.7001, 6.3703) (1.6383, 6.5259) knots 0 0 0 1 2 2 2
  spline S139 degree 2 poles (1.6383, 6.5259) (1.5766, 6.6815) (1.3617, 6.8421) (1.1913, 6.8421) knots 0 0 0 1 2 2 2
  spline S140 degree 2 poles (1.1913, 6.8421) (1.0208, 6.8421) (0.801, 6.6815) (0.7368, 6.521) knots 0 0 0 1 2 2 2
  spline S141 degree 2 poles (0.7368, 6.521) (0.675, 6.3653) (0.6306, 5.8911) (0.6306, 5.5922) knots 0 0 0 1 2 2 2
  spline S142 degree 2 poles (0.6306, 5.5922) (0.6306, 5.2711) (0.6701, 4.8413) (0.7343, 4.6734) knots 0 0 0 1 2 2 2
  spline S143 degree 2 poles (0.7343, 4.6734) (0.7936, 4.5153) (1.0134, 4.3449) (1.1913, 4.3449) knots 0 0 0 1 2 2 2
  spline S144 degree 2 poles (1.1913, 4.3449) (1.3592, 4.3449) (1.579, 4.5054) (1.6408, 4.666) knots 0 0 0 1 2 2 2
  spline S145 degree 2 poles (3.476, 4.0015) (3.2488, 4.0015) (2.8758, 4.1374) (2.7449, 4.2634) knots 0 0 0 1 2 2 2
  spline S146 degree 2 poles (2.7449, 4.2634) (2.6165, 4.3869) (2.4831, 4.7228) (2.4831, 4.913) knots 0 0 0 1 2 2 2
  spline S147 degree 2 poles (2.4831, 4.913) (2.4831, 5.16) (2.7474, 5.5749) (2.9993, 5.6984) knots 0 0 0 1 2 2 2
  line L213 (2.9993, 5.6984) -> (2.9993, 5.7108)
  spline S148 degree 2 poles (2.9993, 5.7108) (2.7745, 5.8417) (2.5572, 6.1529) (2.5572, 6.3851) knots 0 0 0 1 2 2 2
  spline S149 degree 2 poles (2.5572, 6.3851) (2.5572, 6.7284) (3.0759, 7.1879) (3.476, 7.1879) knots 0 0 0 1 2 2 2
  spline S150 degree 2 poles (3.476, 7.1879) (3.891, 7.1879) (4.3924, 6.7531) (4.3924, 6.4123) knots 0 0 0 1 2 2 2
  spline S151 degree 2 poles (4.3924, 6.4123) (4.3924, 6.2073) (4.1528, 5.8071) (3.928, 5.6935) knots 0 0 0 1 2 2 2
  line L214 (3.928, 5.6935) -> (3.928, 5.6812)
  spline S152 degree 2 poles (3.928, 5.6812) (4.1948, 5.5577) (4.469, 5.202) (4.469, 4.9204) knots 0 0 0 1 2 2 2
  spline S153 degree 2 poles (4.469, 4.9204) (4.469, 4.5301) (3.9009, 4.0015) (3.476, 4.0015) knots 0 0 0 1 2 2 2
  spline S154 degree 2 poles (4.0491, 4.8809) (4.0491, 5.0686) (3.9009, 5.2909) (3.6909, 5.4045) knots 0 0 0 1 2 2 2
  spline S155 degree 2 poles (3.6909, 5.4045) (3.6217, 5.444) (3.3896, 5.5354) (3.2438, 5.5947) knots 0 0 0 1 2 2 2
  spline S156 degree 2 poles (3.2438, 5.5947) (3.0759, 5.4836) (2.8956, 5.1526) (2.8956, 4.9426) knots 0 0 0 1 2 2 2
  spline S157 degree 2 poles (2.8956, 4.9426) (2.8956, 4.666) (3.229, 4.3054) (3.481, 4.3054) knots 0 0 0 1 2 2 2
  spline S158 degree 2 poles (3.481, 4.3054) (3.7378, 4.3054) (4.0491, 4.6141) (4.0491, 4.8809) knots 0 0 0 1 2 2 2
  spline S159 degree 2 poles (3.9922, 6.4073) (3.9922, 6.6123) (3.7181, 6.8865) (3.4735, 6.8865) knots 0 0 0 1 2 2 2
  spline S160 degree 2 poles (3.4735, 6.8865) (3.2512, 6.8865) (2.9672, 6.642) (2.9672, 6.432) knots 0 0 0 1 2 2 2
  spline S161 degree 2 poles (2.9672, 6.432) (2.9672, 6.2814) (3.1129, 6.0714) (3.2587, 5.9874) knots 0 0 0 1 2 2 2
  spline S162 degree 2 poles (3.2587, 5.9874) (3.3204, 5.9529) (3.5822, 5.8318) (3.6884, 5.7972) knots 0 0 0 1 2 2 2
  spline S163 degree 2 poles (3.6884, 5.7972) (3.8663, 5.9331) (3.9922, 6.2221) (3.9922, 6.4073) knots 0 0 0 1 2 2 2
  line L215 (6.1091, 7.2546) -> (4.916, 3.4087)
  line L216 (4.916, 3.4087) -> (4.5702, 3.4087)
  line L217 (4.5702, 3.4087) -> (5.7583, 7.2546)
  line L218 (5.7583, 7.2546) -> (6.1091, 7.2546)
  line L219 (8.1715, 4.0707) -> (6.6846, 4.0707)
  line L220 (6.6846, 4.0707) -> (6.6846, 4.3819)
  line L221 (6.6846, 4.3819) -> (7.2379, 4.3819)
  line L222 (7.2379, 4.3819) -> (7.2379, 6.4246)
  line L223 (7.2379, 6.4246) -> (6.6846, 6.4246)
  line L224 (6.6846, 6.4246) -> (6.6846, 6.7037)
  spline S164 degree 2 poles (6.6846, 6.7037) (6.9983, 6.7037) (7.2947, 6.8816) (7.3144, 7.1286) knots 0 0 0 1 2 2 2
  line L225 (7.3144, 7.1286) -> (7.6306, 7.1286)
  line L226 (7.6306, 7.1286) -> (7.6306, 4.3819)
  line L227 (7.6306, 4.3819) -> (8.1715, 4.3819)
  line L228 (8.1715, 4.3819) -> (8.1715, 4.0707)
  spline S165 degree 2 poles (9.5547, 6.8297) (9.4436, 6.8297) (9.2237, 6.7754) (9.1175, 6.7334) knots 0 0 0 1 2 2 2
  spline S166 degree 2 poles (9.1175, 6.7334) (9.0187, 6.6914) (8.873, 6.6025) (8.8162, 6.5629) knots 0 0 0 1 2 2 2
  line L229 (8.8162, 6.5629) -> (8.7915, 6.5629)
  line L230 (8.7915, 6.5629) -> (8.7915, 6.9952)
  spline S167 degree 2 poles (8.7915, 6.9952) (8.9249, 7.0668) (9.3818, 7.1829) (9.5868, 7.1829) knots 0 0 0 1 2 2 2
  spline S168 degree 2 poles (9.5868, 7.1829) (9.7943, 7.1829) (10.1031, 7.0989) (10.229, 7.01) knots 0 0 0 1 2 2 2
  spline S169 degree 2 poles (10.229, 7.01) (10.3624, 6.9137) (10.5007, 6.6346) (10.5007, 6.4469) knots 0 0 0 1 2 2 2
  spline S170 degree 2 poles (10.5007, 6.4469) (10.5007, 6.1949) (10.1698, 5.8145) (9.9376, 5.7651) knots 0 0 0 1 2 2 2
  line L231 (9.9376, 5.7651) -> (9.9376, 5.7355)
  spline S171 degree 2 poles (9.9376, 5.7355) (10.0339, 5.7157) (10.2537, 5.6268) (10.3476, 5.5379) knots 0 0 0 1 2 2 2
  spline S172 degree 2 poles (10.3476, 5.5379) (10.4415, 5.4514) (10.56, 5.1748) (10.56, 4.9747) knots 0 0 0 1 2 2 2
  spline S173 degree 2 poles (10.56, 4.9747) (10.56, 4.7697) (10.4192, 4.4214) (10.2908, 4.2881) knots 0 0 0 1 2 2 2
  spline S174 degree 2 poles (10.2908, 4.2881) (10.1574, 4.1497) (9.7795, 4.0065) (9.5399, 4.0065) knots 0 0 0 1 2 2 2
  spline S175 degree 2 poles (9.5399, 4.0065) (9.3102, 4.0065) (8.8607, 4.1176) (8.7075, 4.1942) knots 0 0 0 1 2 2 2
  line L232 (8.7075, 4.1942) -> (8.7075, 4.6265)
  line L233 (8.7075, 4.6265) -> (8.7372, 4.6265)
  spline S176 degree 2 poles (8.7372, 4.6265) (8.8656, 4.5326) (9.3003, 4.3597) (9.5152, 4.3597) knots 0 0 0 1 2 2 2
  spline S177 degree 2 poles (9.5152, 4.3597) (9.6412, 4.3597) (9.8931, 4.4387) (9.9771, 4.5301) knots 0 0 0 1 2 2 2
  spline S178 degree 2 poles (9.9771, 4.5301) (10.0586, 4.6215) (10.1451, 4.8389) (10.1451, 5.0044) knots 0 0 0 1 2 2 2
  spline S179 degree 2 poles (10.1451, 5.0044) (10.1451, 5.1699) (10.0487, 5.3847) (9.9623, 5.4465) knots 0 0 0 1 2 2 2
  spline S180 degree 2 poles (9.9623, 5.4465) (9.8758, 5.5083) (9.6412, 5.5552) (9.5029, 5.5552) knots 0 0 0 1 2 2 2
  line L234 (9.5029, 5.5552) -> (9.33, 5.5552)
  line L235 (9.33, 5.5552) -> (9.33, 5.8936)
  line L236 (9.33, 5.8936) -> (9.4658, 5.8936)
  spline S181 degree 2 poles (9.4658, 5.8936) (9.74, 5.8936) (10.0858, 6.1554) (10.0858, 6.4049) knots 0 0 0 1 2 2 2
  spline S182 degree 2 poles (10.0858, 6.4049) (10.0858, 6.521) (9.9969, 6.6864) (9.9252, 6.7358) knots 0 0 0 1 2 2 2
  spline S183 degree 2 poles (9.9252, 6.7358) (9.8487, 6.7877) (9.6609, 6.8297) (9.5547, 6.8297) knots 0 0 0 1 2 2 2
  line L237 (12.2866, 7.2546) -> (11.0935, 3.4087)
  line L238 (11.0935, 3.4087) -> (10.7477, 3.4087)
  line L239 (10.7477, 3.4087) -> (11.9358, 7.2546)
  line L240 (11.9358, 7.2546) -> (12.2866, 7.2546)
  line L241 (14.5022, 4.0707) -> (12.6225, 4.0707)
  line L242 (12.6225, 4.0707) -> (12.6225, 4.503)
  spline S184 degree 2 poles (12.6225, 4.503) (12.825, 4.6931) (13.1856, 5.0464) (13.3586, 5.2365) knots 0 0 0 1 2 2 2
  spline S185 degree 2 poles (13.3586, 5.2365) (13.7068, 5.6194) (13.9612, 6.0788) (13.9612, 6.3234) knots 0 0 0 1 2 2 2
  spline S186 degree 2 poles (13.9612, 6.3234) (13.9612, 6.4518) (13.8822, 6.6445) (13.8106, 6.7062) knots 0 0 0 1 2 2 2
  spline S187 degree 2 poles (13.8106, 6.7062) (13.7389, 6.768) (13.5512, 6.8297) (13.4376, 6.8297) knots 0 0 0 1 2 2 2
  spline S188 degree 2 poles (13.4376, 6.8297) (13.3289, 6.8297) (13.1066, 6.7754) (13.0053, 6.7334) knots 0 0 0 1 2 2 2
  spline S189 degree 2 poles (13.0053, 6.7334) (12.9189, 6.6988) (12.7583, 6.6) (12.7089, 6.5654) knots 0 0 0 1 2 2 2
  line L243 (12.7089, 6.5654) -> (12.6867, 6.5654)
  line L244 (12.6867, 6.5654) -> (12.6867, 7.0001)
  spline S190 degree 2 poles (12.6867, 7.0001) (12.8127, 7.0619) (13.2647, 7.1829) (13.4672, 7.1829) knots 0 0 0 1 2 2 2
  spline S191 degree 2 poles (13.4672, 7.1829) (13.8945, 7.1829) (14.3762, 6.7309) (14.3762, 6.3456) knots 0 0 0 1 2 2 2
  spline S192 degree 2 poles (14.3762, 6.3456) (14.3762, 6.1653) (14.2922, 5.8639) (14.2181, 5.7355) knots 0 0 0 1 2 2 2
  spline S193 degree 2 poles (14.2181, 5.7355) (14.144, 5.6021) (13.9291, 5.3403) (13.8106, 5.2143) knots 0 0 0 1 2 2 2
  spline S194 degree 2 poles (13.8106, 5.2143) (13.6179, 5.0044) (13.1461, 4.5548) (13.0053, 4.4239) knots 0 0 0 1 2 2 2
  line L245 (13.0053, 4.4239) -> (14.5022, 4.4239)
  line L246 (14.5022, 4.4239) -> (14.5022, 4.0707)
  spline S195 degree 2 poles (16.7573, 5.0389) (16.7573, 4.8191) (16.6165, 4.4437) (16.4881, 4.3054) knots 0 0 0 1 2 2 2
  spline S196 degree 2 poles (16.4881, 4.3054) (16.3596, 4.167) (15.9768, 4.0065) (15.7396, 4.0065) knots 0 0 0 1 2 2 2
  spline S197 degree 2 poles (15.7396, 4.0065) (15.5223, 4.0065) (15.0974, 4.1028) (14.9418, 4.1794) knots 0 0 0 1 2 2 2
  line L247 (14.9418, 4.1794) -> (14.9418, 4.6116)
  line L248 (14.9418, 4.6116) -> (14.9715, 4.6116)
  spline S198 degree 2 poles (14.9715, 4.6116) (15.0184, 4.5771) (15.1938, 4.4881) (15.3, 4.4486) knots 0 0 0 1 2 2 2
  spline S199 degree 2 poles (15.3, 4.4486) (15.421, 4.4066) (15.6211, 4.3597) (15.7471, 4.3597) knots 0 0 0 1 2 2 2
  spline S200 degree 2 poles (15.7471, 4.3597) (15.8706, 4.3597) (16.1027, 4.4486) (16.1867, 4.5449) knots 0 0 0 1 2 2 2
  spline S201 degree 2 poles (16.1867, 4.5449) (16.2633, 4.6363) (16.3423, 4.8784) (16.3423, 5.0414) knots 0 0 0 1 2 2 2
  spline S202 degree 2 poles (16.3423, 5.0414) (16.3423, 5.2044) (16.2534, 5.4119) (16.1694, 5.4811) knots 0 0 0 1 2 2 2
  spline S203 degree 2 poles (16.1694, 5.4811) (16.083, 5.5577) (15.8261, 5.6219) (15.6705, 5.6219) knots 0 0 0 1 2 2 2
  spline S204 degree 2 poles (15.6705, 5.6219) (15.5025, 5.6219) (15.1691, 5.57) (15.0678, 5.5478) knots 0 0 0 1 2 2 2
  line L249 (15.0678, 5.5478) -> (15.0678, 7.1187)
  line L250 (15.0678, 7.1187) -> (16.74, 7.1187)
  line L251 (16.74, 7.1187) -> (16.74, 6.7605)
  line L252 (16.74, 6.7605) -> (15.4605, 6.7605)
  line L253 (15.4605, 6.7605) -> (15.4605, 5.9479)
  spline S205 degree 2 poles (15.4605, 5.9479) (15.5346, 5.9578) (15.6779, 5.9652) (15.7372, 5.9652) knots 0 0 0 1 2 2 2
  spline S206 degree 2 poles (15.7372, 5.9652) (15.9718, 5.9652) (16.2954, 5.8886) (16.4436, 5.775) knots 0 0 0 1 2 2 2
  spline S207 degree 2 poles (16.4436, 5.775) (16.5943, 5.6614) (16.7573, 5.3156) (16.7573, 5.0389) knots 0 0 0 1 2 2 2
  point P0 (44, -10)
  dimension "d0" = 115
  dimension "d1" = 115
  constraints: 2 other
extrude "Extrusion3" cut sketch "Sketch6" against normal blind 2
body "Solid1"
